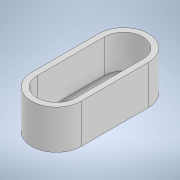
# Autodesk Inventor part: Riel
Saved by Autodesk Inventor 2021 (Build 250183000, 183)
## iProperties
Created: 2021-06-11
Part Number: Riel
Material: Genérico
Document SubType Name: Modeling
Designer: Mecatronica
Density: 1 g/cm^3
Appearance: Valor por defecto
Author: Mecatronica
Autodesk Inventor part; units mm, degrees
ref_plane "YZ Plane" through (0, 0, 0) normal (1, 0, 0) x (0, 1, 0)
ref_plane "XZ Plane" through (0, 0, 0) normal (0, 1, 0) x (-1, 0, 0)
ref_plane "XY Plane" through (0, 0, 0) normal (0, 0, 1) x (1, 0, 0)
sketch "Boceto1" plane through (0, 0, 0) normal (0, 1, 0) x (-1, 0, 0)
  line L0 (22.1667, 30) -> (-22.1667, 30)
  line L1 (-22.1667, 30) -> (-22.1667, -30)
  line L2 (-22.1667, -30) -> (22.1667, -30)
  line L3 (22.1667, -30) -> (22.1667, 30)
  arc A0 (22.1667, 30) -> (-22.1667, 30) centre (0, 30) ccw
  arc A1 (-22.1667, -30) -> (22.1667, -30) centre (0, -30) ccw
  line L4 (17.1667, 30) -> (17.1667, -30)
  line L5 (-17.1667, 30) -> (-17.1667, -30)
  arc A2 (17.1667, 30) -> (-17.1667, 30) centre (0, 30) ccw
  arc A3 (-17.1667, -30) -> (17.1667, -30) centre (0, -30) ccw
  point P0 (0, 0)
  dimension "d0" = 44.3333
  dimension "d1" = 60
  dimension "d2" = 22.1667
  dimension "d3" = 30
  dimension "d4" = 5
  dimension "d5" = 5
  constraints: 12 end point, 8 point on circle, 7 tangent, 5 point on line, 4 centre point, 2 parallel, 2 perpendicular, 1 concentric, 1 horizontal, 1 vertical
  measures "d0" distance between parallel lines of L1 L3
  measures "d1" distance of L0.end L1.end
  measures "d2" distance from line of point (0, 0) L3
  measures "d3" distance from line of point (0, 0) L0
  measures "d4" distance between parallel lines of L3 L4
  measures "d5" distance between parallel lines of L5 L1
extrude "Extrusión1" add sketch "Boceto1" along normal blind 30 contours L3 L2 L4 L0 | L0 A2 A0 | A1 L2 A3 | L0 L5 L2 L1
sketch "Boceto2" plane through (0, 0, 0) normal (0, -1, 0) x (1, 0, 0)
  arc A0 (-22.1667, -30) -> (22.1667, -30) centre (0, -30) ccw projected
  line L0 (-22.1667, -30) -> (-22.1667, 30) projected
  arc A1 (22.1667, 30) -> (-22.1667, 30) centre (0, 30) ccw projected
  line L1 (22.1667, 30) -> (22.1667, -30) projected
  point P0 (0, 0)
extrude "Extrusión2" add sketch "Boceto2" along normal blind 5
equation "\"d2\" = 0.5 * d0"
equation "\"d3\" = 0.5 * d1"
equation "\"d4\" = d5"
